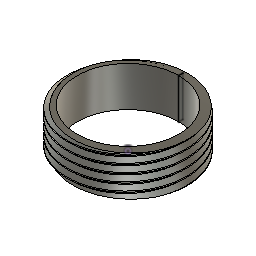
For24mm M30x2 -10mm high - 12.7 radius v1 (Autodesk Fusion 360 design; units mm, degrees)
Autodesk Fusion 360 part; units mm, degrees
note: some values were not read from the file. Chosen so that the rebuilt part matches the saved one: that a step has no effect; where a thread starts. Set by a fixed rule: which sketch regions a step uses.
sketch "Sketch1" plane through (0, 0, 0) normal (1, 0, 0) x (0, 1, 0)
  line L0 (12.7, 0) -> (12.7, 10)
  line L1 (13.7, 10) -> (13.7, 0)
  line L2 (13.7, 0) -> (12.7, 0)
  line L3 (12.7, 10) -> (13.7, 10)
  dimension "d1" = 1
  dimension "d2" = 10
  dimension "d4" = 10
  dimension "d5" = 12.7
  constraint vertical L0
  constraint horizontal L2
  constraint coincident origin L2
  constraint perpendicular L1 L3
  measures "d1" distance of L0.start L1.end
  measures "d2" distance of L0.start L0.end
  measures "d4" distance of L1.start L1.end
  measures "d5" distance of origin L0.start
revolve "Revolve1" add sketch "Sketch1" angle 360 about axis through (0, 0, 1.75) along (0, 0, 1)
thread "Thread1" "ANSI Metric M Profile 30.0 M30x2 6g" major diameter 29.822 minor diameter 27.529 pitch 2 angle 60 modelled right hand crest width 0.2818 on face at (0.6829, 13.683, 6.6667) crest through (0, 14.911, 0.5)
extrude "Extrude4" [no effect]
